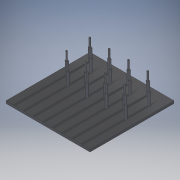
# Autodesk Inventor part: Palma
Saved by Autodesk Inventor 2018 (Build 220112000, 112)
## iProperties
Created: 2017-06-01
Part Number: Palma
Material: Genérico
Document SubType Name: Modeling
Designer: Vitor
Density: 1 g/cm^3
Appearance: Padrão
Author: Vitor
Autodesk Inventor part; units mm, degrees
ref_plane "YZ Plane" through (0, 0, 0) normal (1, 0, 0) x (0, 1, 0)
ref_plane "XZ Plane" through (0, 0, 0) normal (0, 1, 0) x (-1, 0, 0)
ref_plane "XY Plane" through (0, 0, 0) normal (0, 0, 1) x (1, 0, 0)
sketch "Esboço1" plane through (0, 0, 0) normal (0, 0, 1) x (1, 0, 0)
  line L0 (0, 0) -> (100, 0)
  line L1 (100, 0) -> (100, -100)
  line L2 (100, -100) -> (0, -100)
  line L3 (0, -100) -> (0, 0)
  dimension "d0" = 100
  dimension "d1" = 100
  constraints: 8 end point, 2 parallel, 1 horizontal, 1 perpendicular
  measures "d0" distance of L1.end L2.end
  measures "d1" distance of L0.end L1.end
extrude "Extrusão1" add sketch "Esboço1" along normal blind 3
sketch "Esboço2" plane through (0, 0, 3) normal (0, 0, 1) x (1, 0, 0)
  line L0 (0, 0) -> (0, -100) projected
  line L1 (0, 0) -> (9.75, 0)
  line L2 (100, 0) -> (0, 0) projected
  line L3 (9.75, 0) -> (9.75, -10)
  line L4 (9.75, 0) -> (21.25, 0)
  line L5 (21.25, 0) -> (32.75, 0)
  line L6 (32.75, 0) -> (44.25, 0)
  line L7 (44.25, 0) -> (55.75, 0)
  line L8 (55.75, 0) -> (67.25, 0)
  line L9 (67.25, 0) -> (78.75, 0)
  line L10 (78.75, 0) -> (90.25, 0)
  line L11 (90.25, 0) -> (100, 0)
  line L12 (21.25, 0) -> (21.25, -10)
  line L13 (9.75, -10) -> (9.75, -37.6)
  line L14 (9.75, -37.6) -> (21.25, -37.6)
  line L15 (21.25, -37.6) -> (32.75, -37.6)
  line L16 (32.75, -37.6) -> (44.25, -37.6)
  line L17 (44.25, -37.6) -> (55.75, -37.6)
  line L18 (55.75, -37.6) -> (67.25, -37.6)
  line L19 (67.25, -37.6) -> (78.75, -37.6)
  line L20 (78.75, -37.6) -> (90.25, -37.6)
  line L21 (90.25, -37.6) -> (90.25, -10)
  line L22 (90.25, -10) -> (78.75, -10)
  line L23 (78.75, -10) -> (67.25, -10)
  line L24 (67.25, -10) -> (55.75, -10)
  line L25 (55.75, -10) -> (44.25, -10)
  line L26 (44.25, -10) -> (32.75, -10)
  line L27 (32.75, -10) -> (21.25, -10)
  circle A0 centre (9.75, -10) radius 1.5
  circle A1 centre (9.75, -37.6) radius 1.5
  circle A2 centre (32.75, -10) radius 1.5
  circle A3 centre (55.75, -10) radius 1.5
  circle A4 centre (78.75, -10) radius 1.5
  circle A5 centre (78.75, -37.6) radius 1.5
  circle A6 centre (55.75, -37.6) radius 1.5
  circle A7 centre (32.75, -37.6) radius 1.5
  line L28 (21.25, -10) -> (21.25, -20)
  circle A8 centre (21.25, -20) radius 1.5
  line L29 (21.25, -20) -> (21.25, -47.6)
  line L30 (21.25, -47.6) -> (44.25, -47.6)
  line L31 (44.25, -47.6) -> (67.25, -47.6)
  line L32 (67.25, -47.6) -> (90.25, -47.6)
  line L33 (90.25, -47.6) -> (90.25, -20)
  line L34 (90.25, -20) -> (67.25, -20)
  line L35 (67.25, -20) -> (44.25, -20)
  circle A9 centre (21.25, -47.6) radius 1.5
  circle A10 centre (44.25, -47.6) radius 1.5
  circle A11 centre (67.25, -47.6) radius 1.5
  circle A12 centre (90.25, -47.6) radius 1.5
  circle A13 centre (90.25, -20) radius 1.5
  circle A14 centre (67.25, -20) radius 1.5
  circle A15 centre (44.25, -20) radius 1.5
  dimension "d4" = 9.75
  dimension "d5" = 10
  dimension "d7" = 11.5
  dimension "d8" = 11.5
  dimension "d9" = 11.5
  dimension "d10" = 11.5
  dimension "d11" = 11.5
  dimension "d12" = 11.5
  dimension "d13" = 11.5
  dimension "d14" = 27.6
  dimension "d16" = 3
  dimension "d17" = 3
  dimension "d19" = 3
  dimension "d21" = 3
  dimension "d23" = 3
  dimension "d26" = 3
  dimension "d28" = 3
  dimension "d30" = 3
  dimension "d101" = 10
  dimension "d102" = 3
  dimension "d103" = 27.6
  dimension "d104" = 23
  dimension "d105" = 23
  dimension "d106" = 23
  dimension "d107" = 27.6
  dimension "d108" = 23
  dimension "d109" = 23
  dimension "d110" = 3
  dimension "d111" = 3
  dimension "d112" = 3
  dimension "d113" = 3
  dimension "d114" = 3
  dimension "d115" = 3
  dimension "d116" = 3
  constraints: 68 end point, 17 coincident, 16 centre point, 14 point on line, 5 perpendicular, 4 vertical, 2 horizontal, 1 collinear, 9 other
  measures "d4" distance of L0.start L1.end
  measures "d5" distance of L1.end L3.end
  measures "d7" distance of L1.end L4.end
  measures "d8" distance of L4.end L5.end
  measures "d9" distance of L5.end L6.end
  measures "d10" distance of L6.end L7.end
  measures "d11" distance of L7.end L8.end
  measures "d12" distance of L8.end L9.end
  measures "d13" distance of L9.end L10.end
  measures "d14" distance of L13.start L13.end
  measures "d16" diameter of A0
  measures "d17" diameter of A1
  measures "d19" diameter of A2
  measures "d21" diameter of A3
  measures "d23" diameter of A4
  measures "d26" diameter of A5
  measures "d28" diameter of A6
  measures "d30" diameter of A7
  measures "d101" distance of L12.end L28.end
  measures "d102" diameter of A8
  measures "d103" distance of L29.start L29.end
  measures "d104" distance of L29.end L30.end
  measures "d105" distance of L30.end L31.end
  measures "d106" distance of L31.end L32.end
  measures "d107" distance of L32.end L33.end
  measures "d108" distance of L33.end L34.end
  measures "d109" distance of L34.end L35.end
  measures "d110" diameter of A9
  measures "d111" diameter of A10
  measures "d112" diameter of A11
  measures "d113" diameter of A12
  measures "d114" diameter of A13
  measures "d115" diameter of A14
  measures "d116" diameter of A15
extrude "Extrusão6" add sketch "Esboço2" along normal blind 15 contours A15 | A14 L35 L34 | L34 L35 A14 | A0 L13 L3 | L3 L13 A0 | A2 L26 L27 | L27 L26 A2 | A8 L29 L28 | L28 L29 A8 | A1 L14 L13 | L13 L14 A1 | A3 L24 L25 | L25 L24 A3 | A7 L16 L15 | L15 L16 A7 | A9 L30 L29 | L29 L30 A9 | A10 L31 L30 | L30 L31 A10 | A4 L22 L23 | L23 L22 A4 | A6 L18 L17 | L17 L18 A6 | A11 L32 L31 | L31 L32 A11 | A13 L21 | L21 L34 A13 | A5 L20 L19 | L19 L20 A5 | A12 L33 L32 | L32 L33 A12 | L21 A13 L34
sketch "Esboço5" plane through (9.75, -10, 18) normal (0, 0, 1) x (1, 0, 0)
  circle A0 centre (0, 0) radius 1.5 projected
  line L0 (0, 0) -> (23, 0)
  line L1 (23, 0) -> (46, 0)
  line L2 (46, 0) -> (69, 0)
  line L3 (0, 0) -> (0, -27.6)
  line L4 (0, -27.6) -> (23, -27.6)
  line L5 (23, -27.6) -> (46, -27.6)
  line L6 (46, -27.6) -> (69, -27.6)
  line L7 (0, 0) -> (11.5, 0)
  line L8 (11.5, 0) -> (11.5, -10)
  line L9 (11.5, -10) -> (34.5, -10)
  line L10 (34.5, -10) -> (57.5, -10)
  line L11 (57.5, -10) -> (80.5, -10)
  line L12 (80.5, -10) -> (80.5, -37.6)
  line L13 (80.5, -37.6) -> (57.5, -37.6)
  line L14 (57.5, -37.6) -> (34.5, -37.6)
  circle A1 centre (34.5, -37.6) radius 1.5 projected
  line L15 (34.5, -37.6) -> (11.5, -37.6)
  circle A2 centre (0, 0) radius 0.95
  circle A3 centre (11.5, -10) radius 0.95
  circle A4 centre (23, 0) radius 1.5 projected
  circle A5 centre (23, 0) radius 0.95
  circle A6 centre (34.5, -10) radius 0.95
  circle A7 centre (46, 0) radius 1.5 projected
  circle A8 centre (46, 0) radius 0.95
  circle A9 centre (57.5, -10) radius 0.95
  circle A10 centre (69, 0) radius 1.5 projected
  circle A11 centre (69, 0) radius 0.95
  circle A12 centre (80.5, -10) radius 0.95
  circle A13 centre (69, -27.6) radius 0.95
  circle A14 centre (80.5, -37.6) radius 0.95
  circle A15 centre (57.5, -37.6) radius 0.95
  circle A16 centre (46, -27.6) radius 0.95
  circle A17 centre (34.5, -37.6) radius 0.95
  circle A18 centre (23, -27.6) radius 0.95
  circle A19 centre (11.5, -37.6) radius 0.95
  circle A20 centre (0, -27.6) radius 0.95
  point P0 (-9.75, 10)
  dimension "d119" = 23
  dimension "d120" = 23
  dimension "d121" = 23
  dimension "d122" = 27.6
  dimension "d123" = 23
  dimension "d124" = 23
  dimension "d125" = 23
  dimension "d126" = 11.5
  dimension "d127" = 10
  dimension "d128" = 23
  dimension "d129" = 23
  dimension "d130" = 23
  dimension "d131" = 27.6
  dimension "d132" = 23
  dimension "d133" = 23
  dimension "d134" = 23
  constraints: 32 end point, 16 centre point, 16 coincident, 7 point on line, 5 perpendicular, 2 horizontal, 1 midpoint, 1 vertical
  measures "d119" distance of L0.start L0.end
  measures "d120" distance of L0.end L1.end
  measures "d121" distance of L1.end L2.end
  measures "d122" distance of L0.start L3.end
  measures "d123" distance of L3.end L4.end
  measures "d124" distance of L4.end L5.end
  measures "d125" distance of L5.end L6.end
  measures "d126" distance of L0.start L7.end
  measures "d127" distance of L7.end L8.end
  measures "d128" distance of L8.end L9.end
  measures "d129" distance of L9.end L10.end
  measures "d130" distance of L10.end L11.end
  measures "d131" distance of L11.end L12.end
  measures "d132" distance of L12.end L13.end
  measures "d133" distance of L13.end L14.end
  measures "d134" distance of L15.start L15.end
extrude "Extrusão7" add sketch "Esboço5" along normal blind 10 contours A13 | A16 L6 L5 | L5 L6 A16 | A18 L5 L4 | L4 L5 A18 | A20 L4 L3 | L3 L4 A20 | A11 | A19 | A15 L14 L13 | L13 L14 A15 | A14 L13 L12 | L12 L13 A14 | A12 L12 L11 | L11 L12 A12 | A9 L11 L10 | L10 L11 A9 | A6 L10 L9 | L9 L10 A6 | A3 L9 L8 | L8 L9 A3 | A2 L3 L0 | L0 L3 A2 | A5 L1 L0 | L0 L1 A5 | A8 L2 L1 | L1 L2 A8 | A17 L15 L14 | L14 L15 A17
